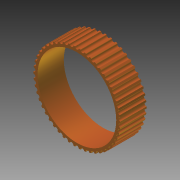
# Autodesk Inventor part: new wheel rim
Saved by Autodesk Inventor 2012 (Build 160160000, 160)
## iProperties
Created: 2012-08-10
Part Number: new wheel rim
Material: Default
Document SubType Name: Modeling
Designer: Bryce
Density: 1 g/cm^3
Author: Bryce
Autodesk Inventor part; units mm, degrees
ref_plane "YZ Plane" through (0, 0, 0) normal (1, 0, 0) x (0, 1, 0)
ref_plane "XZ Plane" through (0, 0, 0) normal (0, 1, 0) x (-1, 0, 0)
ref_plane "XY Plane" through (0, 0, 0) normal (0, 0, 1) x (1, 0, 0)
sketch "Sketch1" plane through (0, 0, 0) normal (0, 0, 1) x (1, 0, 0)
  circle A0 centre (0, 0) radius 33.3375
  arc A1 (-1.5871, 36.7958) -> (0, 35.2425) centre (0, 36.83) ccw
  line L0 (0, 36.83) -> (0, 0) construction
  arc A2 (0, 35.2425) -> (1.5871, 36.7958) centre (0, 36.83) ccw
  arc A3 (-6.1864, 36.3067) -> (-4.4171, 34.9646) centre (-4.616, 36.5396) ccw
  arc A4 (-4.4171, 34.9646) -> (-3.0371, 36.7046) centre (-4.616, 36.5396) ccw
  arc A5 (-10.688, 35.2451) -> (-8.7645, 34.1353) centre (-9.1592, 35.6729) ccw
  arc A6 (-8.7645, 34.1353) -> (-7.6135, 36.0345) centre (-9.1592, 35.6729) ccw
  arc A7 (-15.0211, 33.6276) -> (-12.9736, 32.7676) centre (-13.558, 34.2437) ccw
  arc A8 (-12.9736, 32.7676) -> (-12.0698, 34.7961) centre (-13.558, 34.2437) ccw
  arc A9 (-19.1173, 31.4798) -> (-16.9782, 30.8832) centre (-17.743, 32.2744) ccw
  arc A10 (-16.9782, 30.8832) -> (-16.3357, 33.009) centre (-17.743, 32.2744) ccw
  arc A11 (-22.912, 28.8355) -> (-20.715, 28.5118) centre (-21.6481, 29.7961) ccw
  arc A12 (-20.715, 28.5118) -> (-20.344, 30.7013) centre (-21.6481, 29.7961) ccw
  arc A13 (-26.3454, 25.7365) -> (-24.1252, 25.6907) centre (-25.2119, 26.8479) ccw
  arc A14 (-24.1252, 25.6907) -> (-24.0315, 27.9094) centre (-25.2119, 26.8479) ccw
  arc A15 (-29.3633, 22.2316) -> (-27.1548, 22.4644) centre (-28.378, 23.4763) ccw
  arc A16 (-27.1548, 22.4644) -> (-27.34, 24.6774) centre (-28.378, 23.4763) ccw
  arc A17 (-31.9181, 18.3761) -> (-29.7562, 18.8839) centre (-31.0966, 19.7345) ccw
  arc A18 (-29.7562, 18.8839) -> (-30.2173, 21.0562) centre (-31.0966, 19.7345) ccw
  arc A19 (-33.9696, 14.2308) -> (-31.8884, 15.0055) centre (-33.3248, 15.6815) ccw
  arc A20 (-31.8884, 15.0055) -> (-32.6181, 17.103) centre (-33.3248, 15.6815) ccw
  arc A21 (-35.4853, 9.8611) -> (-33.5176, 10.8905) centre (-35.0274, 11.3811) ccw
  arc A22 (-33.5176, 10.8905) -> (-34.5044, 12.88) centre (-35.0274, 11.3811) ccw
  arc A23 (-36.4414, 5.3358) -> (-34.6183, 6.6038) centre (-36.1776, 6.9013) ccw
  arc A24 (-34.6183, 6.6038) -> (-35.8466, 8.4539) centre (-36.1776, 6.9013) ccw
  arc A25 (-36.8228, 0.7264) -> (-35.173, 2.2129) centre (-36.7573, 2.3126) ccw
  arc A26 (-35.173, 2.2129) -> (-36.6235, 3.8944) centre (-36.7573, 2.3126) ccw
  arc A27 (-36.6235, -3.8944) -> (-35.173, -2.2129) centre (-36.7573, -2.3126) ccw
  arc A28 (-35.173, -2.2129) -> (-36.8228, -0.7264) centre (-36.7573, -2.3126) ccw
  arc A29 (-35.8466, -8.4539) -> (-34.6183, -6.6038) centre (-36.1776, -6.9013) ccw
  arc A30 (-34.6183, -6.6038) -> (-36.4414, -5.3358) centre (-36.1776, -6.9013) ccw
  arc A31 (-34.5044, -12.88) -> (-33.5176, -10.8905) centre (-35.0274, -11.3811) ccw
  arc A32 (-33.5176, -10.8905) -> (-35.4853, -9.8611) centre (-35.0274, -11.3811) ccw
  arc A33 (-32.6181, -17.103) -> (-31.8884, -15.0055) centre (-33.3248, -15.6815) ccw
  arc A34 (-31.8884, -15.0055) -> (-33.9696, -14.2308) centre (-33.3248, -15.6815) ccw
  arc A35 (-30.2173, -21.0562) -> (-29.7562, -18.8839) centre (-31.0966, -19.7345) ccw
  arc A36 (-29.7562, -18.8839) -> (-31.9181, -18.3761) centre (-31.0966, -19.7345) ccw
  arc A37 (-27.34, -24.6774) -> (-27.1548, -22.4644) centre (-28.378, -23.4763) ccw
  arc A38 (-27.1548, -22.4644) -> (-29.3633, -22.2316) centre (-28.378, -23.4763) ccw
  arc A39 (-24.0315, -27.9094) -> (-24.1252, -25.6907) centre (-25.2119, -26.8479) ccw
  arc A40 (-24.1252, -25.6907) -> (-26.3454, -25.7365) centre (-25.2119, -26.8479) ccw
  arc A41 (-20.344, -30.7013) -> (-20.715, -28.5118) centre (-21.6481, -29.7961) ccw
  arc A42 (-20.715, -28.5118) -> (-22.912, -28.8355) centre (-21.6481, -29.7961) ccw
  arc A43 (-16.3357, -33.009) -> (-16.9782, -30.8832) centre (-17.743, -32.2744) ccw
  arc A44 (-16.9782, -30.8832) -> (-19.1173, -31.4798) centre (-17.743, -32.2744) ccw
  arc A45 (-12.0698, -34.7961) -> (-12.9736, -32.7676) centre (-13.558, -34.2437) ccw
  arc A46 (-12.9736, -32.7676) -> (-15.0211, -33.6276) centre (-13.558, -34.2437) ccw
  arc A47 (-7.6135, -36.0345) -> (-8.7645, -34.1353) centre (-9.1592, -35.6729) ccw
  arc A48 (-8.7645, -34.1353) -> (-10.688, -35.2451) centre (-9.1592, -35.6729) ccw
  arc A49 (-3.0371, -36.7046) -> (-4.4171, -34.9646) centre (-4.616, -36.5396) ccw
  arc A50 (-4.4171, -34.9646) -> (-6.1864, -36.3067) centre (-4.616, -36.5396) ccw
  arc A51 (1.5871, -36.7958) -> (0, -35.2425) centre (0, -36.83) ccw
  arc A52 (0, -35.2425) -> (-1.5871, -36.7958) centre (0, -36.83) ccw
  arc A53 (6.1864, -36.3067) -> (4.4171, -34.9646) centre (4.616, -36.5396) ccw
  arc A54 (4.4171, -34.9646) -> (3.0371, -36.7046) centre (4.616, -36.5396) ccw
  arc A55 (10.688, -35.2451) -> (8.7645, -34.1353) centre (9.1592, -35.6729) ccw
  arc A56 (8.7645, -34.1353) -> (7.6135, -36.0345) centre (9.1592, -35.6729) ccw
  arc A57 (15.0211, -33.6276) -> (12.9736, -32.7676) centre (13.558, -34.2437) ccw
  arc A58 (12.9736, -32.7676) -> (12.0698, -34.7961) centre (13.558, -34.2437) ccw
  arc A59 (19.1173, -31.4798) -> (16.9782, -30.8832) centre (17.743, -32.2744) ccw
  arc A60 (16.9782, -30.8832) -> (16.3357, -33.009) centre (17.743, -32.2744) ccw
  arc A61 (22.912, -28.8355) -> (20.715, -28.5118) centre (21.6481, -29.7961) ccw
  arc A62 (20.715, -28.5118) -> (20.344, -30.7013) centre (21.6481, -29.7961) ccw
  arc A63 (26.3454, -25.7365) -> (24.1252, -25.6907) centre (25.2119, -26.8479) ccw
  arc A64 (24.1252, -25.6907) -> (24.0315, -27.9094) centre (25.2119, -26.8479) ccw
  arc A65 (29.3633, -22.2316) -> (27.1548, -22.4644) centre (28.378, -23.4763) ccw
  arc A66 (27.1548, -22.4644) -> (27.34, -24.6774) centre (28.378, -23.4763) ccw
  arc A67 (31.9181, -18.3761) -> (29.7562, -18.8839) centre (31.0966, -19.7345) ccw
  arc A68 (29.7562, -18.8839) -> (30.2173, -21.0562) centre (31.0966, -19.7345) ccw
  arc A69 (33.9696, -14.2308) -> (31.8884, -15.0055) centre (33.3248, -15.6815) ccw
  arc A70 (31.8884, -15.0055) -> (32.6181, -17.103) centre (33.3248, -15.6815) ccw
  arc A71 (-10.688, 35.2451) -> (-12.0698, 34.7961) centre (0, 0) ccw
  arc A72 (-7.6135, 36.0345) -> (-10.688, 35.2451) centre (0, 0) ccw construction
  arc A73 (-6.1864, 36.3067) -> (-7.6135, 36.0345) centre (0, 0) ccw
  arc A74 (-3.0371, 36.7046) -> (-6.1864, 36.3067) centre (0, 0) ccw construction
  arc A75 (-12.0698, 34.7961) -> (-15.0211, 33.6276) centre (0, 0) ccw construction
  arc A76 (-15.0211, 33.6276) -> (-16.3357, 33.009) centre (0, 0) ccw
  arc A77 (-16.3357, 33.009) -> (-19.1173, 31.4798) centre (0, 0) ccw construction
  arc A78 (-19.1173, 31.4798) -> (-20.344, 30.7013) centre (0, 0) ccw
  arc A79 (-20.344, 30.7013) -> (-22.912, 28.8355) centre (0, 0) ccw construction
  arc A80 (-22.912, 28.8355) -> (-24.0315, 27.9094) centre (0, 0) ccw
  arc A81 (-26.3454, 25.7365) -> (-27.34, 24.6774) centre (0, 0) ccw
  arc A82 (-27.34, 24.6774) -> (-29.3633, 22.2316) centre (0, 0) ccw construction
  arc A83 (-29.3633, 22.2316) -> (-30.2173, 21.0562) centre (0, 0) ccw
  arc A84 (-31.9181, 18.3761) -> (-32.6181, 17.103) centre (0, 0) ccw
  arc A85 (-30.2173, 21.0562) -> (-31.9181, 18.3761) centre (0, 0) ccw construction
  arc A86 (-32.6181, 17.103) -> (-33.9696, 14.2308) centre (0, 0) ccw construction
  arc A87 (-33.9696, 14.2308) -> (-34.5044, 12.88) centre (0, 0) ccw
  arc A88 (-24.0315, 27.9094) -> (-26.3454, 25.7365) centre (0, 0) ccw construction
  arc A89 (-35.4853, 9.8611) -> (-35.8466, 8.4539) centre (0, 0) ccw
  arc A90 (-36.4414, 5.3358) -> (-36.6235, 3.8944) centre (0, 0) ccw
  arc A91 (-36.8228, 0.7264) -> (-36.8228, -0.7264) centre (0, 0) ccw
  arc A92 (-36.6235, 3.8944) -> (-36.8228, 0.7264) centre (0, 0) ccw construction
  arc A93 (-35.8466, 8.4539) -> (-36.4414, 5.3358) centre (0, 0) ccw construction
  arc A94 (-34.5044, 12.88) -> (-35.4853, 9.8611) centre (0, 0) ccw construction
  arc A95 (-36.8228, -0.7264) -> (-36.6235, -3.8944) centre (0, 0) ccw construction
  arc A96 (-36.6235, -3.8944) -> (-36.4414, -5.3358) centre (0, 0) ccw
  arc A97 (-36.4414, -5.3358) -> (-35.8466, -8.4539) centre (0, 0) ccw construction
  arc A98 (-35.8466, -8.4539) -> (-35.4853, -9.8611) centre (0, 0) ccw
  arc A99 (-35.4853, -9.8611) -> (-34.5044, -12.88) centre (0, 0) ccw construction
  arc A100 (-34.5044, -12.88) -> (-33.9696, -14.2308) centre (0, 0) ccw
  arc A101 (-33.9696, -14.2308) -> (-32.6181, -17.103) centre (0, 0) ccw construction
  arc A102 (-32.6181, -17.103) -> (-31.9181, -18.3761) centre (0, 0) ccw
  arc A103 (-31.9181, -18.3761) -> (-30.2173, -21.0562) centre (0, 0) ccw construction
  arc A104 (-30.2173, -21.0562) -> (-29.3633, -22.2316) centre (0, 0) ccw
  arc A105 (-27.34, -24.6774) -> (-26.3454, -25.7365) centre (0, 0) ccw
  arc A106 (-26.3454, -25.7365) -> (-24.0315, -27.9094) centre (0, 0) ccw construction
  arc A107 (-24.0315, -27.9094) -> (-22.912, -28.8355) centre (0, 0) ccw
  arc A108 (-22.912, -28.8355) -> (-20.344, -30.7013) centre (0, 0) ccw construction
  arc A109 (-20.344, -30.7013) -> (-19.1173, -31.4798) centre (0, 0) ccw
  arc A110 (-19.1173, -31.4798) -> (-16.3357, -33.009) centre (0, 0) ccw construction
  arc A111 (-16.3357, -33.009) -> (-15.0211, -33.6276) centre (0, 0) ccw
  arc A112 (-15.0211, -33.6276) -> (-12.0698, -34.7961) centre (0, 0) ccw construction
  arc A113 (-12.0698, -34.7961) -> (-10.688, -35.2451) centre (0, 0) ccw
  arc A114 (-10.688, -35.2451) -> (-7.6135, -36.0345) centre (0, 0) ccw construction
  arc A115 (-7.6135, -36.0345) -> (-6.1864, -36.3067) centre (0, 0) ccw
  arc A116 (-6.1864, -36.3067) -> (-3.0371, -36.7046) centre (0, 0) ccw construction
  arc A117 (-3.0371, -36.7046) -> (-1.5871, -36.7958) centre (0, 0) ccw
  arc A118 (-1.5871, -36.7958) -> (1.5871, -36.7958) centre (0, 0) ccw construction
  arc A119 (1.5871, -36.7958) -> (3.0371, -36.7046) centre (0, 0) ccw
  arc A120 (3.0371, -36.7046) -> (6.1864, -36.3067) centre (0, 0) ccw construction
  arc A121 (6.1864, -36.3067) -> (7.6135, -36.0345) centre (0, 0) ccw
  arc A122 (-29.3633, -22.2316) -> (-27.34, -24.6774) centre (0, 0) ccw construction
  arc A123 (7.6135, -36.0345) -> (10.688, -35.2451) centre (0, 0) ccw construction
  arc A124 (10.688, -35.2451) -> (12.0698, -34.7961) centre (0, 0) ccw
  arc A125 (12.0698, -34.7961) -> (15.0211, -33.6276) centre (0, 0) ccw construction
  arc A126 (16.3357, -33.009) -> (19.1173, -31.4798) centre (0, 0) ccw construction
  arc A127 (19.1173, -31.4798) -> (20.344, -30.7013) centre (0, 0) ccw
  arc A128 (15.0211, -33.6276) -> (16.3357, -33.009) centre (0, 0) ccw
  arc A129 (22.912, -28.8355) -> (24.0315, -27.9094) centre (0, 0) ccw
  arc A130 (20.344, -30.7013) -> (22.912, -28.8355) centre (0, 0) ccw construction
  arc A131 (24.0315, -27.9094) -> (26.3454, -25.7365) centre (0, 0) ccw construction
  arc A132 (26.3454, -25.7365) -> (27.34, -24.6774) centre (0, 0) ccw
  arc A133 (27.34, -24.6774) -> (29.3633, -22.2316) centre (0, 0) ccw construction
  arc A134 (29.3633, -22.2316) -> (30.2173, -21.0562) centre (0, 0) ccw
  arc A135 (30.2173, -21.0562) -> (31.9181, -18.3761) centre (0, 0) ccw construction
  arc A136 (31.9181, -18.3761) -> (32.6181, -17.103) centre (0, 0) ccw
  arc A137 (32.6181, -17.103) -> (33.9696, -14.2308) centre (0, 0) ccw construction
  arc A138 (1.5871, 36.7958) -> (0, 36.83) centre (0, 0) ccw construction
  arc A139 (0, 36.83) -> (-1.5871, 36.7958) centre (0, 0) ccw construction
  arc A140 (-1.5871, 36.7958) -> (-3.0371, 36.7046) centre (0, 0) ccw
  arc A141 (35.4853, -9.8611) -> (33.5176, -10.8905) centre (35.0274, -11.3811) ccw
  arc A142 (33.5176, -10.8905) -> (34.5044, -12.88) centre (35.0274, -11.3811) ccw
  arc A143 (36.4414, -5.3358) -> (34.6183, -6.6038) centre (36.1776, -6.9013) ccw
  arc A144 (34.6183, -6.6038) -> (35.8466, -8.4539) centre (36.1776, -6.9013) ccw
  arc A145 (36.8228, -0.7264) -> (35.173, -2.2129) centre (36.7573, -2.3126) ccw
  arc A146 (35.173, -2.2129) -> (36.6235, -3.8944) centre (36.7573, -2.3126) ccw
  arc A147 (36.6235, 3.8944) -> (35.173, 2.2129) centre (36.7573, 2.3126) ccw
  arc A148 (35.173, 2.2129) -> (36.8228, 0.7264) centre (36.7573, 2.3126) ccw
  arc A149 (35.8466, 8.4539) -> (34.6183, 6.6038) centre (36.1776, 6.9013) ccw
  arc A150 (34.6183, 6.6038) -> (36.4414, 5.3358) centre (36.1776, 6.9013) ccw
  arc A151 (34.5044, 12.88) -> (33.5176, 10.8905) centre (35.0274, 11.3811) ccw
  arc A152 (33.5176, 10.8905) -> (35.4853, 9.8611) centre (35.0274, 11.3811) ccw
  arc A153 (32.6181, 17.103) -> (31.8884, 15.0055) centre (33.3248, 15.6815) ccw
  arc A154 (31.8884, 15.0055) -> (33.9696, 14.2308) centre (33.3248, 15.6815) ccw
  arc A155 (30.2173, 21.0562) -> (29.7562, 18.8839) centre (31.0966, 19.7345) ccw
  arc A156 (29.7562, 18.8839) -> (31.9181, 18.3761) centre (31.0966, 19.7345) ccw
  arc A157 (27.34, 24.6774) -> (27.1548, 22.4644) centre (28.378, 23.4763) ccw
  arc A158 (27.1548, 22.4644) -> (29.3633, 22.2316) centre (28.378, 23.4763) ccw
  arc A159 (24.0315, 27.9094) -> (24.1252, 25.6907) centre (25.2119, 26.8479) ccw
  arc A160 (24.1252, 25.6907) -> (26.3454, 25.7365) centre (25.2119, 26.8479) ccw
  arc A161 (20.344, 30.7013) -> (20.715, 28.5118) centre (21.6481, 29.7961) ccw
  arc A162 (20.715, 28.5118) -> (22.912, 28.8355) centre (21.6481, 29.7961) ccw
  arc A163 (16.3357, 33.009) -> (16.9782, 30.8832) centre (17.743, 32.2744) ccw
  arc A164 (16.9782, 30.8832) -> (19.1173, 31.4798) centre (17.743, 32.2744) ccw
  arc A165 (12.0698, 34.7961) -> (12.9736, 32.7676) centre (13.558, 34.2437) ccw
  arc A166 (12.9736, 32.7676) -> (15.0211, 33.6276) centre (13.558, 34.2437) ccw
  arc A167 (7.6135, 36.0345) -> (8.7645, 34.1353) centre (9.1592, 35.6729) ccw
  arc A168 (8.7645, 34.1353) -> (10.688, 35.2451) centre (9.1592, 35.6729) ccw
  arc A169 (3.0371, 36.7046) -> (4.4171, 34.9646) centre (4.616, 36.5396) ccw
  arc A170 (4.4171, 34.9646) -> (6.1864, 36.3067) centre (4.616, 36.5396) ccw
  arc A171 (3.0371, 36.7046) -> (1.5871, 36.7958) centre (0, 0) ccw
  arc A172 (7.6135, 36.0345) -> (6.1864, 36.3067) centre (0, 0) ccw
  arc A173 (12.0698, 34.7961) -> (10.688, 35.2451) centre (0, 0) ccw
  arc A174 (16.3357, 33.009) -> (15.0211, 33.6276) centre (0, 0) ccw
  arc A175 (20.344, 30.7013) -> (19.1173, 31.4798) centre (0, 0) ccw
  arc A176 (24.0315, 27.9094) -> (22.912, 28.8355) centre (0, 0) ccw
  arc A177 (27.34, 24.6774) -> (26.3454, 25.7365) centre (0, 0) ccw
  arc A178 (30.2173, 21.0562) -> (29.3633, 22.2316) centre (0, 0) ccw
  arc A179 (32.6181, 17.103) -> (31.9181, 18.3761) centre (0, 0) ccw
  arc A180 (34.5044, 12.88) -> (33.9696, 14.2308) centre (0, 0) ccw
  arc A181 (35.8466, 8.4539) -> (35.4853, 9.8611) centre (0, 0) ccw
  arc A182 (36.6235, 3.8944) -> (36.4414, 5.3358) centre (0, 0) ccw
  arc A183 (36.8228, -0.7264) -> (36.8228, 0.7264) centre (0, 0) ccw
  arc A184 (36.4414, -5.3358) -> (36.6235, -3.8944) centre (0, 0) ccw
  arc A185 (33.9696, -14.2308) -> (34.5044, -12.88) centre (0, 0) ccw
  arc A186 (35.4853, -9.8611) -> (35.8466, -8.4539) centre (0, 0) ccw
  dimension "d10" = 73.66
  dimension "d0" = 66.675
  dimension "d1" = 36.83
  dimension "d5" = 360
  dimension "d17" = 1.5875
  constraints: 198 point on circle, 100 centre point, 4 vertical alignment, 2 end point, 2 point on line, 1 coincident, 1 horizontal alignment, 1 line through centre, 1 vertical, 558 other
  measures "d0" diameter of A0
  measures "d1" distance of point (0, 0) L0.start
  measures "d17" radius of A2
extrude "Extrusion1" add sketch "Sketch1" along normal blind 22.225
equation "\"d1\" = 0.5 * d10"
body "Solid1"
